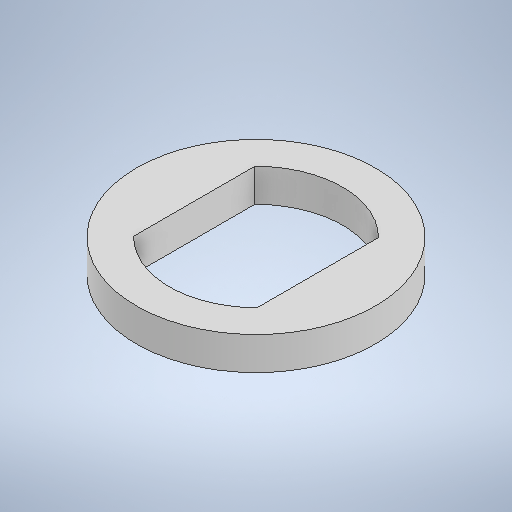
# Autodesk Inventor part: LoadCellFitting
Saved by Autodesk Inventor 2025.2 (Build 292293000, 293)
## iProperties
Created: 2025-09-23
Part Number: LoadCellFitting
Material: Generic
Document SubType Name: Modeling
Designer: Simon
Density: 1 g/cm^3
Appearance: Default
Author: Simon
Autodesk Inventor part; units mm, degrees
ref_plane "YZ Plane" through (0, 0, 0) normal (1, 0, 0) x (0, 1, 0)
ref_plane "XZ Plane" through (0, 0, 0) normal (0, 1, 0) x (-1, 0, 0)
ref_plane "XY Plane" through (0, 0, 0) normal (0, 0, 1) x (1, 0, 0)
sketch "Sketch1" plane through (0, 0, 0) normal (0, 1, 0) x (-1, 0, 0)
  circle A0 centre (0, 0) radius 14.5
  circle A1 centre (0, 0) radius 10.5
  line L0 (14.5, 0) -> (7.5, 0)
  line L1 (-14.5, 0) -> (-7.5, 0)
  line L2 (7.5, -7.3485) -> (7.5, 7.3485)
  line L3 (-7.5, -7.3485) -> (-7.5, 7.3485)
  dimension "d0" = 29
  dimension "d1" = 21
  dimension "d2" = 7
  dimension "d3" = 7
  constraints: 8 end point, 4 point on circle, 2 centre point, 2 coincident, 2 horizontal, 2 midpoint, 1 parallel, 1 vertical
  measures "d0" diameter of A0
  measures "d1" diameter of A1
  measures "d2" distance of L0.start L0.end
  measures "d3" distance of L1.start L1.end
extrude "Extrusion1" add sketch "Sketch1" along normal blind 4 contours L0 A1 L1 A0 | A0 L1 A1 L0 | L0 L2 A1 | A1 L2 L0 | L1 L3 A1 | A1 L3 L1
body "Solid1"
